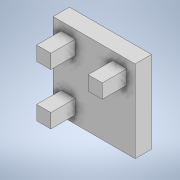
# Autodesk Inventor part: final_beam_cube_top
Saved by Autodesk Inventor 2021 (Build 250183000, 183)
## iProperties
Created: 2021-06-14
Part Number: final_beam_cube_top
Material: Generic
Document SubType Name: Modeling
Designer: user
Density: 1 g/cm^3
Appearance: Default
Author: user
Autodesk Inventor part; units mm, degrees
ref_plane "YZ Plane" through (0, 0, 0) normal (1, 0, 0) x (0, 1, 0)
ref_plane "XZ Plane" through (0, 0, 0) normal (0, 1, 0) x (-1, 0, 0)
ref_plane "XY Plane" through (0, 0, 0) normal (0, 0, 1) x (1, 0, 0)
sketch "Sketch1" plane through (0, 0, 0) normal (0, 0, 1) x (1, 0, 0)
  line L0 (-22.7093, 18.0885) -> (27.2907, 18.0885)
  line L1 (27.2907, 18.0885) -> (27.2907, -31.9115)
  line L2 (27.2907, -31.9115) -> (-22.7093, -31.9115)
  line L3 (-22.7093, -31.9115) -> (-22.7093, 18.0885)
  point P0 (0, 0)
  dimension "d0" = 50
  dimension "d1" = 50
  constraints: 8 end point, 2 parallel, 1 horizontal, 1 perpendicular
  measures "d0" distance of L0.start L0.end
  measures "d1" distance of L2.end L0.start
extrude "Extrusion1" add sketch "Sketch1" along normal blind 10
sketch "Sketch3" plane through (0, 0, 10) normal (0, 0, 1) x (1, 0, 0)
  line L0 (-17.7093, 13.0885) -> (-9.0593, 13.0885)
  line L1 (-9.0593, 13.0885) -> (-9.0593, 4.4385)
  line L2 (-9.0593, 4.4385) -> (-17.7093, 4.4385)
  line L3 (-17.7093, 4.4385) -> (-17.7093, 13.0885)
  line L4 (-22.7093, 18.0885) -> (-22.7093, -31.9115) projected
  line L5 (27.2907, 18.0885) -> (-22.7093, 18.0885) projected
  line L6 (13.6407, 13.0885) -> (22.2907, 13.0885)
  line L7 (22.2907, 13.0885) -> (22.2907, 4.4385)
  line L8 (22.2907, 4.4385) -> (13.6407, 4.4385)
  line L9 (13.6407, 4.4385) -> (13.6407, 13.0885)
  line L10 (-17.7093, -18.2615) -> (-9.0593, -18.2615)
  line L11 (-9.0593, -18.2615) -> (-9.0593, -26.9115)
  line L12 (-9.0593, -26.9115) -> (-17.7093, -26.9115)
  line L13 (-17.7093, -26.9115) -> (-17.7093, -18.2615)
  line L14 (27.2907, -31.9115) -> (27.2907, 18.0885) projected
  line L15 (-22.7093, -31.9115) -> (27.2907, -31.9115) projected
  point P0 (0, 0)
  dimension "d8" = 5
  dimension "d9" = 5
  dimension "d10" = 8.65
  dimension "d11" = 8.65
  dimension "d12" = 5
  dimension "d13" = 8.65
  dimension "d14" = 8.65
  dimension "d15" = 5
  dimension "d16" = 5
  dimension "d17" = 5
  dimension "d18" = 8.65
  dimension "d19" = 8.65
  constraints: 24 end point, 6 parallel, 3 horizontal, 3 perpendicular
  measures "d8" distance between parallel lines of L4 L3
  measures "d9" distance between parallel lines of L5 L0
  measures "d10" distance of L0.end L1.end
  measures "d11" distance of L1.end L2.end
  measures "d12" distance between parallel lines of L5 L6
  measures "d13" distance of L7.end L8.end
  measures "d14" distance of L8.end L6.start
  measures "d15" distance between parallel lines of L14 L7
  measures "d16" distance between parallel lines of L15 L12
  measures "d17" distance between parallel lines of L4 L13
  measures "d18" distance of L10.start L10.end
  measures "d19" distance of L10.end L11.end
extrude "Extrusion2" add sketch "Sketch3" along normal blind 15 contours L0 L1 L2 L3 | L6 L7 L8 L9 | L10 L11 L12 L13
equation "\"d13\" = d10"
equation "\"d15\" = d12"
equation "\"d16\" = d8"
equation "\"d19\" = d18"
body "Solid1"
